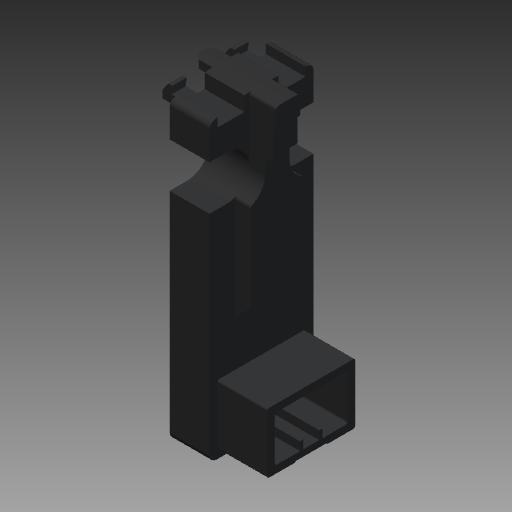
# Autodesk Inventor part: 3779382 VUVG-LK-IP40
Saved by Autodesk Inventor 2017.1 (Build 211199000, 199)
## iProperties
Category: PARTsolutions
Company: FESTO
Created: 2016-12-21
Part Number: 3779382 VUVG-LK-IP40
Catalog Web Link: www.cadenas.de
Description: VUVG IP40-Cover
Vendor: FESTO
Document SubType Name: Modeling
Designer: psAdmin
Manufacturer: FESTO
Mass: 0.638888 g
Surface Area: 13.2696 cm^2
Volume: 0.638888 cm^3
Density: 1 g/cm^3
Material: Generic
Appearance: PSOLRGB-80-80-80
PSOL_IDENT_0: {$CADENAS_DATA\23d-libs\festo\parts\v\vuvg\parts\vuvg_lk_ip40.prj},185 {VTYP=3D},{NB=3779382 VUVG-LK
PSOL_IDENT_1: -IP40},{LINA=3779382 VUVG-LK-IP40},{NN=VUVG IP40},{DATE=21.01.2016 17:00:12},{GEOMDATE=21.01.2016 16
PSOL_IDENT_2: :23:00},{VERSION=},{LINEID=10},{LINESUBID=-1},{WBVAR=}  {NB=3779382 VUVG-LK-IP40},{LINA=3779382 VUVG
PSOL_IDENT_3: -LK-IP40},{KT=DUMMY},{TNR=3779382},{TYP=VUVG-LK-IP40}
NN: VUVG IP40
NT: Cover
NB: 3779382 VUVG-LK-IP40
NBSYN: $TNR. $TYP.
LINA: 3779382 VUVG-LK-IP40
TNR: 3779382
TYP: VUVG-LK-IP40
SUPPLIER: FESTO
ARTICLENO: 3779382 VUVG-LK-IP40
BOMINFO: 3779382 VUVG-LK-IP40
CREATOR: CADENAS GmbH
Title: 3779382 VUVG-LK-IP40
Author: Cadenas PARTsolutions
Comments: Cover
Autodesk Inventor part; units mm, degrees
sketch "Sketch_1" plane through (0, 0, 0) normal (1, 0, 0) x (0, 1, 0)
  arc A0 (0.7, 4.9) -> (0, 4.2) centre (0.7, 4.2) ccw
  line L0 (0, 4.2) -> (0, -4.2)
  arc A1 (0, -4.2) -> (0.7, -4.9) centre (0.7, -4.2) ccw
  line L1 (0.7, -4.9) -> (27.3163, -4.9)
  arc A2 (27.3163, -4.9) -> (27.7927, -4.5517) centre (27.3163, -4.4) ccw
  arc A3 (27.7927, -4.5517) -> (27.7927, 4.5517) centre (13.5, 0) ccw
  arc A4 (27.7927, 4.5517) -> (27.3163, 4.9) centre (27.3163, 4.4) ccw
  line L2 (27.3163, 4.9) -> (0.7, 4.9)
  constraints: 10 point on circle, 6 end point, 5 centre point
extrude "Extrusion1" add sketch "Sketch_1" along normal blind 8.45
sketch "Sketch_2" plane through (3.75, 0, 0) normal (1, 0, 0) x (0, 0, -1)
  line L0 (-6, 29) -> (-6, -1)
  line L1 (-6, -1) -> (6, -1)
  line L2 (6, -1) -> (6, 29)
  line L3 (6, 29) -> (-6, 29)
  line L4 (-4.15, 6.25) -> (-4.15, 0.95)
  arc A0 (-4.15, 0.95) -> (-3.95, 0.75) centre (-3.95, 0.95) ccw
  line L5 (-3.95, 0.75) -> (3.95, 0.75)
  arc A1 (3.95, 0.75) -> (4.15, 0.95) centre (3.95, 0.95) ccw
  line L6 (4.15, 0.95) -> (4.15, 6.25)
  arc A2 (4.15, 6.25) -> (3.95, 6.45) centre (3.95, 6.25) ccw
  line L7 (3.95, 6.45) -> (-3.95, 6.45)
  arc A3 (-3.95, 6.45) -> (-4.15, 6.25) centre (-3.95, 6.25) ccw
  constraints: 16 end point, 8 point on circle, 4 centre point
extrude "Extrusion2" cut sketch "Sketch_2" along normal blind 8.45
sketch "Sketch_3" plane through (3.75, 0, 0) normal (1, 0, 0) x (0, 0, -1)
  line L0 (-3.45, 5.55) -> (-3.45, 1.65)
  arc A0 (-3.45, 1.65) -> (-3.25, 1.45) centre (-3.25, 1.65) ccw
  line L1 (-3.25, 1.45) -> (-1.05, 1.45)
  line L2 (-1.05, 1.45) -> (-1.05, 2.25)
  line L3 (-1.05, 2.25) -> (-0.75, 2.25)
  line L4 (-0.75, 2.25) -> (-0.75, 1.45)
  line L5 (-0.75, 1.45) -> (0.75, 1.45)
  line L6 (0.75, 1.45) -> (0.75, 2.25)
  line L7 (0.75, 2.25) -> (1.05, 2.25)
  line L8 (1.05, 2.25) -> (1.05, 1.45)
  line L9 (1.05, 1.45) -> (3.25, 1.45)
  arc A1 (3.25, 1.45) -> (3.45, 1.65) centre (3.25, 1.65) ccw
  line L10 (3.45, 1.65) -> (3.45, 5.55)
  arc A2 (3.45, 5.55) -> (3.25, 5.75) centre (3.25, 5.55) ccw
  line L11 (3.25, 5.75) -> (-3.25, 5.75)
  arc A3 (-3.25, 5.75) -> (-3.45, 5.55) centre (-3.25, 5.55) ccw
  constraints: 24 end point, 8 point on circle, 4 centre point
extrude "Extrusion3" cut sketch "Sketch_3" along normal blind 8.45
sketch "Sketch_4" plane through (3.75, 0, 0) normal (1, 0, 0) x (0, 0, -1)
  line L0 (1.6, 5.05) -> (1.6, 3.15)
  line L1 (1.6, 3.15) -> (2.4, 3.15)
  line L2 (2.4, 3.15) -> (2.4, 5.05)
  line L3 (2.4, 5.05) -> (1.6, 5.05)
  constraints: 8 end point
extrude "Extrusion4" cut sketch "Sketch_4" against normal blind 8.45
sketch "Sketch_5" plane through (3.75, 0, 0) normal (1, 0, 0) x (0, 0, -1)
  line L0 (-2.4, 5.05) -> (-2.4, 3.15)
  line L1 (-2.4, 3.15) -> (-1.6, 3.15)
  line L2 (-1.6, 3.15) -> (-1.6, 5.05)
  line L3 (-1.6, 5.05) -> (-2.4, 5.05)
  constraints: 8 end point
extrude "Extrusion5" cut sketch "Sketch_5" against normal blind 8.45
sketch "Sketch_7" plane through (3.75, 0, 0) normal (1, 0, 0) x (0, 0, -1)
  line L0 (-2.5, 20.3419) -> (-2.5, 10.775)
  line L1 (-2.5, 10.775) -> (2.5, 10.775)
  line L2 (2.5, 10.775) -> (2.5, 20.3419)
  arc A0 (2.5, 20.3419) -> (2.3312, 20.6116) centre (2.2, 20.3419) ccw
  arc A1 (1.15, 22.5) -> (2.3312, 20.6116) centre (3.25, 22.5) ccw
  line L3 (1.15, 22.5) -> (1.15, 28.1754)
  arc A2 (1.15, 28.1754) -> (0.8673, 28.4749) centre (0.85, 28.1754) ccw
  arc A3 (0.8673, 28.4749) -> (-0.8673, 28.4749) centre (0, 13.5) ccw
  arc A4 (-0.8673, 28.4749) -> (-1.15, 28.1754) centre (-0.85, 28.1754) ccw
  line L4 (-1.15, 28.1754) -> (-1.15, 22.5)
  arc A5 (-2.3312, 20.6116) -> (-1.15, 22.5) centre (-3.25, 22.5) ccw
  arc A6 (-2.3312, 20.6116) -> (-2.5, 20.3419) centre (-2.2, 20.3419) ccw
  constraints: 14 point on circle, 10 end point, 7 centre point
extrude "Extrusion6" add sketch "Sketch_7" along normal blind 2.5
sketch "Sketch_8" plane through (0, 0, 0) normal (0, 0, 1) x (1, 0, 0)
  line L0 (3.75, 10.775) -> (11.25, 10.775)
  line L1 (11.25, 10.775) -> (11.25, 30.775)
  line L2 (11.25, 30.775) -> (6.25, 30.775)
  line L3 (6.25, 30.775) -> (6.25, 26.65)
  line L4 (6.25, 26.65) -> (6, 26.4)
  line L5 (6, 26.4) -> (6, 24.25)
  line L6 (6, 24.25) -> (5.25, 23.5)
  line L7 (5.25, 23.5) -> (5.25, 12.275)
  line L8 (5.25, 12.275) -> (3.75, 10.775)
  constraints: 18 end point
extrude "Extrusion7" cut sketch "Sketch_8" along normal mid plane 6
sketch "Sketch_6" plane through (3.75, 0, 0) normal (1, 0, 0) x (0, 0, -1)
  line L0 (-7, 20.4) -> (-3.25, 20.4)
  arc A0 (-3.25, 20.4) -> (-3.25, 24.6) centre (-3.25, 22.5) ccw
  line L1 (-3.25, 24.6) -> (-6, 24.6)
  line L2 (-6, 24.6) -> (-6, 30.06)
  line L3 (-6, 30.06) -> (-4.15, 30.06)
  line L4 (-4.15, 30.06) -> (-4.15, 27.06)
  line L5 (-4.15, 27.06) -> (-1.6, 27.06)
  line L6 (-1.6, 27.06) -> (-1.6, 29.06)
  line L7 (-1.6, 29.06) -> (1.6, 29.06)
  line L8 (1.6, 29.06) -> (1.6, 27.06)
  line L9 (1.6, 27.06) -> (4.15, 27.06)
  line L10 (4.15, 27.06) -> (4.15, 30.06)
  line L11 (4.15, 30.06) -> (6, 30.06)
  line L12 (6, 30.06) -> (6, 24.6)
  line L13 (6, 24.6) -> (3.25, 24.6)
  arc A1 (3.25, 24.6) -> (3.25, 20.4) centre (3.25, 22.5) ccw
  line L14 (3.25, 20.4) -> (7, 20.4)
  line L15 (7, 20.4) -> (7, 31.06)
  line L16 (7, 31.06) -> (-7, 31.06)
  line L17 (-7, 31.06) -> (-7, 20.4)
  constraints: 36 end point, 4 point on circle, 2 centre point
extrude "Extrusion8" cut sketch "Sketch_6" along normal mid plane 10
sketch "Sketch_9" plane through (0, 0, 0) normal (1, 0, 0) x (0, 1, 0)
  line L0 (19.25, 4.15) -> (0.75, 4.15)
  line L1 (0.75, 4.15) -> (0.75, -4.15)
  line L2 (0.75, -4.15) -> (19.25, -4.15)
  line L3 (19.25, -4.15) -> (19.25, 4.15)
  constraints: 8 end point
extrude "Extrusion9" cut sketch "Sketch_9" along normal blind 3
sketch "Sketch_13" plane through (0, 0, 0) normal (0, 0, 1) x (1, 0, 0)
  line L0 (-1.97, 27.06) -> (-1.97, 26.31)
  line L1 (-1.97, 26.31) -> (0, 26.31)
  line L2 (0, 26.31) -> (0, 27.06)
  line L3 (0, 27.06) -> (-1.0487, 27.06)
  arc A0 (-1.1469, 27.1791) -> (-1.0487, 27.06) centre (-1.0487, 27.16) ccw
  line L4 (-1.1469, 27.1791) -> (-1.0358, 27.7505)
  arc A1 (-1.0358, 27.7505) -> (-1.0849, 27.81) centre (-1.0849, 27.76) ccw
  line L5 (-1.0849, 27.81) -> (-1.3232, 27.81)
  arc A2 (-1.3232, 27.81) -> (-1.485, 27.7276) centre (-1.3232, 27.61) ccw
  line L6 (-1.485, 27.7276) -> (-1.97, 27.06)
  constraints: 14 end point, 6 point on circle, 3 centre point
extrude "Extrusion10" add sketch "Sketch_13" along normal mid plane 7.2
sketch "Sketch_14" plane through (0, 0, 0) normal (0, 1, 0) x (-1, 0, 0)
  line L0 (3, 2.25) -> (0, 2.25)
  line L1 (0, 2.25) -> (0, -2.25)
  line L2 (0, -2.25) -> (3, -2.25)
  line L3 (3, -2.25) -> (3, 2.25)
  constraints: 8 end point
extrude "Extrusion11" cut sketch "Sketch_14" along normal blind 30
sketch "Sketch_11" plane through (0, 0, 0) normal (1, 0, 0) x (0, 1, 0)
  line L0 (28.4745, 0.875) -> (27.7231, 0.875)
  arc A0 (27.7231, -0.875) -> (27.7231, 0.875) centre (13.5, 0) ccw
  line L1 (27.7231, -0.875) -> (28.4745, -0.875)
  arc A1 (28.4745, -0.875) -> (28.4745, 0.875) centre (13.5, 0) ccw
  constraints: 4 end point, 4 point on circle, 2 centre point
extrude "Extrusion12" add sketch "Sketch_11" against normal blind 1.85
sketch "Sketch_10" plane through (0, 0, 0) normal (0, 1, 0) x (-1, 0, 0)
  line L0 (3.85, 0.875) -> (1.2843, 0.875)
  line L1 (1.2843, 0.875) -> (1.85, 0.3093)
  line L2 (1.85, 0.3093) -> (1.85, -0.3093)
  line L3 (1.85, -0.3093) -> (1.2843, -0.875)
  line L4 (1.2843, -0.875) -> (3.85, -0.875)
  line L5 (3.85, -0.875) -> (3.85, 0.875)
  constraints: 12 end point
extrude "Extrusion13" cut sketch "Sketch_10" along normal blind 30
sketch "Sketch_12" plane through (0, 0, 0) normal (0, 1, 0) x (-1, 0, 0)
  line L0 (-1.1, -1.2) -> (-1.1, 1.2)
  arc A0 (-1.1, 1.2) -> (-1.4, 1.5) centre (-1.4, 1.2) ccw
  line L1 (-1.4, 1.5) -> (-9.1, 1.5)
  line L2 (-9.1, 1.5) -> (-9.1, -1.5)
  line L3 (-9.1, -1.5) -> (-1.4, -1.5)
  arc A1 (-1.4, -1.5) -> (-1.1, -1.2) centre (-1.4, -1.2) ccw
  constraints: 8 end point, 4 point on circle, 2 centre point
extrude "Extrusion14" cut sketch "Sketch_12" along normal blind 0.85
ref_plane "NEBV_XY" through (5.296, 4.1, 0) normal (1, 0, 0) x (0, 0, 1)
ref_plane "NEBV_YZ" through (5.296, 4.1, 0) normal (0, 0, 1) x (0, -1, 0)
ref_plane "NEBV_ZX" through (5.296, 4.1, 0) normal (0, -1, 0) x (1, 0, 0)
ref_plane "VAVE_XY" through (0.92, 0.2, 0) normal (0, -1, 0) x (1, 0, 0)
ref_plane "VAVE_YZ" through (0.92, 0.2, 0) normal (1, 0, 0) x (0, 0, 1)
ref_plane "VAVE_ZX" through (0.92, 0.2, 0) normal (0, 0, 1) x (0, -1, 0)
body "Solid1"
